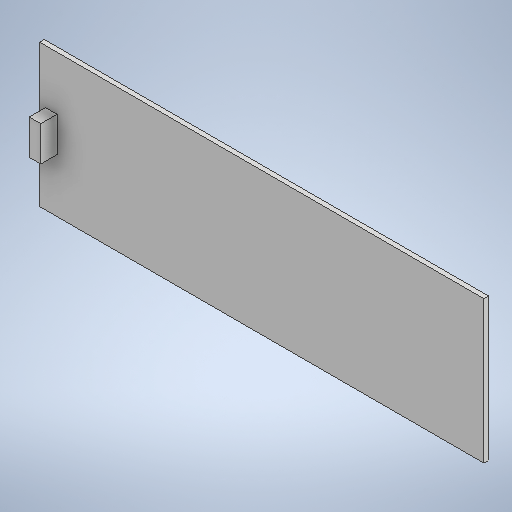
# Autodesk Inventor part: Door
Saved by Autodesk Inventor 2025.2 (Build 292293000, 293)
## iProperties
Created: 2025-04-05
Part Number: Door
Material: Generic
Document SubType Name: Modeling
Designer: pipep
Density: 1 g/cm^3
Appearance: Default
Author: pipep
Autodesk Inventor part; units mm, degrees
ref_plane "YZ Plane" through (0, 0, 0) normal (1, 0, 0) x (0, 1, 0)
ref_plane "XZ Plane" through (0, 0, 0) normal (0, 1, 0) x (-1, 0, 0)
ref_plane "XY Plane" through (0, 0, 0) normal (0, 0, 1) x (1, 0, 0)
sketch "Sketch1" plane through (0, 0, 0) normal (0, 1, 0) x (-1, 0, 0)
  point P0 (0, 0)
sketch "Sketch6" plane through (0, 0, 0) normal (0, 0, 1) x (1, 0, 0)
  line L0 (0, 0) -> (184, 0)
  line L1 (184, 0) -> (184, 61.2)
  line L2 (184, 61.2) -> (0, 61.2)
  line L3 (0, 61.2) -> (0, 0)
  line L4 (0, 0) -> (184, 0)
  line L5 (184, 0) -> (184, 61.2)
  dimension "d18" = 184
  dimension "d19" = 61.2
  constraints: 12 end point, 2 horizontal, 2 parallel, 1 perpendicular, 1 vertical
  measures "d18" distance of L0.start L0.end
  measures "d19" distance of L0.end L1.end
extrude "Extrusion5" add sketch "Sketch6" along normal blind 2
sketch "Sketch7" plane through (0, 0, 2) normal (0, 0, 1) x (1, 0, 0)
  line L0 (184, 61.2) -> (0, 61.2) projected
  line L1 (0, 61.2) -> (0, 30.6)
  line L2 (0, 30.6) -> (2.5, 30.6)
  line L3 (2.5, 30.6) -> (2.5, 38.1)
  line L4 (2.5, 30.6) -> (2.5, 23.1)
  line L5 (2.5, 38.1) -> (7.5, 38.1)
  line L6 (7.5, 38.1) -> (7.5, 23.1)
  line L7 (7.5, 23.1) -> (2.5, 23.1)
  point P0 (0, 0)
  dimension "d22" = 30.6
  dimension "d23" = 2.5
  dimension "d24" = 7.5
  dimension "d25" = 7.5
  dimension "d26" = 5
  constraints: 14 end point, 3 perpendicular, 2 horizontal, 2 vertical
  measures "d22" distance of L0.end L1.end
  measures "d23" distance of L1.end L2.end
  measures "d24" distance of L2.end L3.end
  measures "d25" distance of L2.end L4.end
  measures "d26" distance of L3.end L5.end
extrude "Extrusion6" add sketch "Sketch7" along normal blind 7
sketch "Sketch8" plane through (0, 0, 2) normal (0, 0, 1) x (1, 0, 0)
  line L0 (184, 61.2) -> (0, 61.2) projected
  line L1 (184, 61.2) -> (191, 61.2)
  line L2 (191, 61.2) -> (191, 0)
  line L3 (191, 0) -> (184, 0)
  line L4 (184, 0) -> (184, 61.2)
  point P0 (0, 0)
  dimension "d29" = 7
  constraints: 8 end point, 2 parallel, 1 horizontal, 1 perpendicular
  measures "d29" distance of L2.end L3.end
extrude "Extrusion7" add sketch "Sketch8" against normal blind 2
sketch "Sketch2" plane through (0, 0, 0) normal (0, 1, 0) x (-1, 0, 0)
  line L0 (0, 0) -> (92.58, 0)
  line L1 (92.58, 0) -> (92.58, -29.35)
  line L2 (92.58, -29.35) -> (0, -29.35)
  line L3 (0, -29.35) -> (0, 29.35)
  line L4 (0, 29.35) -> (92.58, 29.35)
  line L5 (92.58, 29.35) -> (92.58, -29.35)
  dimension "d0" = 92.58
  dimension "d1" = 29.35
  dimension "d2" = 92.58
  dimension "d3" = 58.7
  constraints: 12 end point, 2 horizontal, 2 parallel, 2 perpendicular
  measures "d0" distance of L0.start L0.end
  measures "d1" distance of L0.end L1.end
  measures "d2" distance of L3.end L4.end
  measures "d3" distance of L2.end L3.end
sketch "Sketch3" plane through (0, 3, 0) normal (0, 1, 0) x (1, 0, 0)
  line L0 (0, 0) -> (-10, 0)
  line L1 (-10, 0) -> (-10, 7.5)
  line L2 (-10, 7.5) -> (-15, 7.5)
  line L3 (-15, 7.5) -> (-15, -7.5)
  line L4 (-15, -7.5) -> (-10, -7.5)
  line L5 (-10, -7.5) -> (-10, 7.5)
  dimension "d6" = 10
  dimension "d7" = 7.5
  dimension "d8" = 5
  dimension "d9" = 15
  constraints: 12 end point, 2 horizontal, 2 parallel, 2 perpendicular
  measures "d6" distance of L0.start L0.end
  measures "d7" distance of L0.end L1.end
  measures "d8" distance of L4.end L3.end
  measures "d9" distance of L3.end L2.end
sketch "Sketch4" plane through (0, 3, 0) normal (0, 1, 0) x (1, 0, 0)
  line L0 (0, -29.35) -> (0, 29.35) projected
  line L1 (0, -29.35) -> (0, -34.35)
  line L2 (0, -34.35) -> (-5, -34.35)
  line L3 (-5, -34.35) -> (-5, -29.35)
  line L4 (-92.58, -29.35) -> (0, -29.35) projected
  line L5 (-5, -29.35) -> (0, -29.35)
  point P0 (0, 0)
  dimension "d12" = 5
  dimension "d13" = 5
  constraints: 8 end point, 2 perpendicular, 1 horizontal, 1 vertical
  measures "d12" distance of L0.start L1.end
  measures "d13" distance of L1.end L2.end
sketch "Sketch5" plane through (0, 8, 0) normal (0, 1, 0) x (1, 0, 0)
  line L0 (-15, 7.5) -> (-15, -7.5) projected
  line L1 (-10, -7.5) -> (-10, 7.5) projected
  line L2 (-15, 7.5) -> (-10, 7.5)
  line L3 (-10, 7.5) -> (-10, -7.5)
  line L4 (-10, -7.5) -> (-15, -7.5)
  line L5 (-15, -7.5) -> (-15, 7.5)
  point P0 (0, 0)
  constraints: 8 end point, 2 parallel, 1 horizontal, 1 perpendicular
equation "\"d2\" = d0"
equation "\"d3\" = 2 * d1"
equation "\"d9\" = 2 * d7"
body "Solid1"
body "Solid2"
